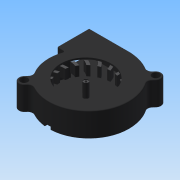
# Autodesk Inventor part: 5015 kuler obduva ulitla
Saved by Autodesk Inventor 2017 (Build 210142000, 142)
## iProperties
Part Number: 5015 kuler obduva ulitla
Material: Типовые
Document SubType Name: Modeling
Designer: alcapone
Density: 1 g/cm^3
Appearance: Резина — черная
Mass: 8.81297 g
Surface Area: 142.043 cm^2
Volume: 8.81297 cm^3
Author: alcapone
Autodesk Inventor part; units mm, degrees
ref_plane "YZ Plane" through (0, 0, 0) normal (1, 0, 0) x (0, 1, 0)
ref_plane "XZ Plane" through (0, 0, 0) normal (0, 1, 0) x (-1, 0, 0)
ref_plane "XY Plane" through (0, 0, 0) normal (0, 0, 1) x (1, 0, 0)
sketch "Эскиз1" plane through (0, 0, 0) normal (0, 0, 1) x (1, 0, 0)
  circle A0 centre (0, 0) radius 13
  circle A1 centre (0, 0) radius 15.5
  circle A2 centre (-18, -20) radius 2.25
  circle A3 centre (20, 23) radius 2.25
  line L0 (-25.4, 27.55) -> (-25.4, 7.95)
  line L1 (-25.4, 7.95) -> (-22, 7.95)
  line L2 (-25.4, 27.55) -> (0, 27.55)
  line L3 (25.6, 31.451287) -> (25.6, -25.798713) construction
  arc A4 (22.43532, 20.847857) -> (17.56468, 25.152143) centre (20, 23) ccw
  arc A5 (-20.43532, -17.847857) -> (-15.56468, -22.152143) centre (-18, -20) ccw
  line L4 (17.56468, 25.152143) -> (16.739143, 24.217982)
  line L5 (-19.151802, -16.395455) -> (-20.43532, -17.847857)
  line L6 (21.282046, 19.542837) -> (22.43532, 20.847857)
  line L7 (-15.56468, -22.152143) -> (-14.81527, -21.304126)
  line L8 (-54, -23.75) -> (48, -23.75) construction
  arc A6 (-11.116766, -20.664695) -> (25.6, 1) centre (0.85, 1) ccw
  arc A7 (-21.05304, 6.62865) -> (-18.846796, -12.833353) centre (0.718164, -0.759385) ccw
  arc A8 (-21.05304, 6.62865) -> (-22, 7.95) centre (-22, 6.95) ccw
  arc A9 (-19.151802, -16.395455) -> (-18.846796, -12.833353) centre (-21.399789, -14.408862) ccw
  arc A10 (-11.116766, -20.664695) -> (-14.81527, -21.304126) centre (-12.567283, -23.290719) ccw
  arc A11 (25.6, 1) -> (21.044444, 15.876409) centre (-0.967627, 1) ccw
  arc A12 (12.922672, 23.64726) -> (0, 27.55) centre (-0.967627, 1) ccw
  arc A13 (12.922672, 23.64726) -> (16.739143, 24.217982) centre (14.491156, 26.204575) ccw
  arc A14 (21.282046, 19.542837) -> (21.044444, 15.876409) centre (23.530033, 17.556244) ccw
  line L9 (-25.4, 26.2) -> (1.943816, 26.2)
  line L10 (-25.4, 9.3) -> (-18.611597, 9.3)
  arc A15 (-18.611597, 9.3) -> (0.782803, -22.549904) centre (0.718164, -0.759385) ccw
  arc A16 (0.782803, -22.549904) -> (24.4, 1) centre (0.85, 1) ccw
  arc A17 (24.4, 1) -> (1.943816, 26.2) centre (-0.967627, 1) ccw
  line L11 (-25.4, 27.55) -> (-25.4, 26.2)
  line L12 (-25.4, 9.3) -> (-25.4, 7.95)
  point P0 (-20.558936, 7.95)
  point P1 (14.991388, 22.24026)
  point P2 (-17.605238, -14.645396)
  point P3 (19.675218, 17.724585)
  point P4 (-13.144564, -19.41359)
  dimension "d0" = 26
  dimension "d1" = 31
  dimension "d2" = 4.5
  dimension "d3" = 4.5
  dimension "d4" = 20
  dimension "d5" = 18
  dimension "d6" = 20
  dimension "d7" = 23
  dimension "d8" = 25.4
  dimension "d9" = 25.4
  dimension "d10" = 51
  dimension "d12" = 19.6
  dimension "d13" = 6.5
  dimension "d14" = 6.5
  dimension "d16" = 25.6
  dimension "d17" = 51.3
  dimension "d18" = 0.5
  dimension "d19" = 1
  dimension "d20" = 22
  dimension "d21" = 3
  dimension "d22" = 3
  dimension "d23" = 22.99062
  dimension "d24" = 24.75
  dimension "d25" = 3
  dimension "d26" = 26.56763
  dimension "d27" = 26.56763
  dimension "d28" = 1.35
  dimension "d29" = 1.35
  dimension "d30" = 1.2
  dimension "d31" = 1.2
  dimension "d32" = 1.2
  dimension "d133" = 90
  dimension "d138" = 16.9
  constraints: 33 point on circle, 26 end point, 20 tangent, 18 centre point, 8 point on line, 7 coincident, 3 parallel, 2 collinear, 2 horizontal, 2 perpendicular, 2 vertical, 1 equal radius
  measures "d0" diameter of A0
  measures "d1" diameter of A1
  measures "d2" diameter of A2
  measures "d3" diameter of A3
  measures "d4" vertical distance of A2.centre A1.centre
  measures "d5" horizontal distance of point (0, 0) A2.centre
  measures "d6" horizontal distance of point (0, 0) A3.centre
  measures "d7" vertical distance of A3.centre point (0, 0)
  measures "d8" distance from line of point (0, 0) L0
  measures "d9" distance of L0.start L2.end
  measures "d10" distance between parallel lines of L0 L3
  measures "d12" distance between parallel lines of L1 L2
  measures "d13" diameter of A4
  measures "d14" diameter of A5
  measures "d16" distance from line of L3 point (0, 0)
  measures "d17" distance between parallel lines of L8 L2
  measures "d18" distance edge to line of A5 L8
  measures "d19" radius of A8
  measures "d20" horizontal distance of point (0, 0) A8.centre
  measures "d21" radius of A9
  measures "d22" radius of A10
  measures "d23" radius of A7
  measures "d24" radius of A6
  measures "d25" radius of A13
  measures "d26" radius of A12
  measures "d27" radius of A11
  measures "d28" distance between parallel lines of L9 L2
  measures "d29" distance between parallel lines of L10 L1
  measures "d30" radial gap between concentric circles of A7 A15
  measures "d31" radial gap between concentric circles of A6 A16
  measures "d32" radial gap between concentric circles of A12 A17
  measures "d133" angle of L2 L0
  measures "d138" distance between parallel lines of L10 L9
sketch "Эскиз1 outline for Выдавливание1" plane through (0, 0, 0) normal (0, 0, 1) x (1, 0, 0)
  line L0 (0, 27.55) -> (-25.4, 27.55)
  line L1 (-25.4, 27.55) -> (-25.4, 7.95)
  line L2 (-25.4, 7.95) -> (-22, 7.95)
  arc A0 (-22, 7.95) -> (-21.05304, 6.62865) centre (-22, 6.95) cw
  arc A1 (-21.05304, 6.62865) -> (-18.846796, -12.833353) centre (0.718164, -0.759385) ccw
  arc A2 (-18.846796, -12.833353) -> (-19.151802, -16.395455) centre (-21.399789, -14.408862) cw
  line L3 (-19.151802, -16.395455) -> (-20.43532, -17.847857)
  arc A3 (-20.43532, -17.847857) -> (-15.56468, -22.152143) centre (-18, -20) ccw
  line L4 (-15.56468, -22.152143) -> (-14.81527, -21.304126)
  arc A4 (-14.81527, -21.304126) -> (-11.116766, -20.664695) centre (-12.567283, -23.290719) cw
  arc A5 (-11.116766, -20.664695) -> (25.6, 1) centre (0.85, 1) ccw
  arc A6 (25.6, 1) -> (21.044444, 15.876409) centre (-0.967627, 1) ccw
  arc A7 (21.044444, 15.876409) -> (21.282046, 19.542837) centre (23.530033, 17.556244) cw
  line L5 (21.282046, 19.542837) -> (22.43532, 20.847857)
  arc A8 (22.43532, 20.847857) -> (17.56468, 25.152143) centre (20, 23) ccw
  line L6 (17.56468, 25.152143) -> (16.739143, 24.217982)
  arc A9 (16.739143, 24.217982) -> (12.922672, 23.64726) centre (14.491156, 26.204575) cw
  arc A10 (12.922672, 23.64726) -> (0, 27.55) centre (-0.967627, 1) ccw
  circle A11 centre (-18, -20) radius 2.25
  circle A12 centre (20, 23) radius 2.25
  circle A13 centre (0, 0) radius 15.5
extrude "Выдавливание1" add sketch "Эскиз1 outline for Выдавливание1" along normal mid plane 15
sketch "Эскиз1 outline for Выдавливание2" plane through (0, 0, 0) normal (0, 0, 1) x (1, 0, 0)
  circle A0 centre (0, 0) radius 15.5
extrude "Выдавливание2" add sketch "Эскиз1 outline for Выдавливание2" against normal blind 7.5
sketch "Эскиз1 outline for Выдавливание3" plane through (0, 0, 0) normal (0, 0, 1) x (1, 0, 0)
  line L0 (1.943816, 26.2) -> (-25.4, 26.2)
  arc A0 (24.4, 1) -> (1.943816, 26.2) centre (-0.967627, 1) ccw
  arc A1 (0.782803, -22.549904) -> (24.4, 1) centre (0.85, 1) ccw
  arc A2 (-18.611597, 9.3) -> (0.782803, -22.549904) centre (0.718164, -0.759385) ccw
  line L1 (-25.4, 9.3) -> (-18.611597, 9.3)
  line L2 (-25.4, 26.2) -> (-25.4, 9.3)
extrude "Выдавливание3" cut sketch "Эскиз1 outline for Выдавливание3" along normal blind 6.5 and the other way blind 6.2
sketch "Эскиз2" plane through (0, 0, -7.5) normal (0, 0, -1) x (-1, 0, 0)
  line L0 (0, 0) -> (0, 39) construction
  arc A0 (2, -8.774964) -> (-2, -8.774964) centre (0, 0) ccw
  arc A1 (-1.943816, 26.2) -> (-24.4, 1) centre (0.967627, 1) ccw
  arc A2 (-24.4, 1) -> (-0.782803, -22.549904) centre (-0.85, 1) ccw
  arc A3 (-0.782803, -22.549904) -> (18.611597, 9.3) centre (-0.718164, -0.759385) ccw
  arc A4 (-22.887217, 9.629191) -> (-24.4, 1) centre (0.967627, 1) ccw
  line L1 (-2, -20) -> (1, -20)
  line L2 (1, -20) -> (1, -18.276492)
  line L3 (1, -18.276492) -> (-2, -18.276492)
  line L4 (-3, -22.451652) -> (-3, -9.539392)
  line L5 (3, -9.539392) -> (3, -22.230439)
  line L6 (-2, -8.774964) -> (-2, -18.276492)
  line L7 (-2, -20) -> (-2, -22.521905)
  line L8 (2, -22.379803) -> (2, -8.774964)
  arc A5 (-2, -22.521905) -> (2, -22.376912) centre (-0.85, 1) ccw
  line L9 (-0.8, 9.967949) -> (-0.8, 24.420616)
  line L10 (0.8, 24.293495) -> (0.8, 9.967949)
  line L11 (0, 0) -> (-32, 0) construction
  line L12 (0, 0) -> (28, 0) construction
  line L13 (0, 0.533734) -> (-31.257467, 31.7912) construction
  line L14 (0, 0) -> (-29.841247, -29.841247) construction
  arc A6 (-0.8, 9.967949) -> (-6.189332, 7.854436) centre (0, 0) ccw
  line L15 (-24.399212, 0.8) -> (-9.967949, 0.8)
  line L16 (-9.967949, -0.8) -> (-24.331109, -0.8)
  line L17 (9.967949, 0.8) -> (21.028696, 0.8)
  line L18 (10.072158, -0.8) -> (21.072413, -0.8)
  line L19 (6.482719, 7.614089) -> (15.385181, 16.516552)
  line L20 (-15.944824, -17.076194) -> (-6.482719, -7.614089)
  line L21 (7.614089, 6.482719) -> (16.394183, 15.262812)
  arc A7 (9.967949, 0.8) -> (7.614089, 6.482719) centre (0, 0) ccw
  arc A8 (6.482719, 7.614089) -> (0.8, 9.967949) centre (0, 0) ccw
  arc A9 (-6.482719, -7.614089) -> (-3, -9.539392) centre (0, 0) ccw
  arc A10 (-7.36357, 6.765932) -> (-9.967949, 0.8) centre (0, 0) ccw
  arc A11 (-9.967949, -0.8) -> (-7.614089, -6.482719) centre (0, 0) ccw
  line L22 (-17.139173, -16.007802) -> (-7.614089, -6.482719)
  arc A12 (3, -9.539392) -> (6.765932, -7.36357) centre (0, 0) ccw
  arc A13 (7.986272, -6.189332) -> (10.072158, -0.8) centre (0, 0) ccw
  line L23 (-16.909631, 18.574735) -> (-6.189332, 7.854436)
  line L24 (7.986272, -6.189332) -> (16.24014, -14.4432)
  line L25 (15.123801, -15.721438) -> (6.765932, -7.36357)
  line L26 (-7.36357, 6.765932) -> (-18.052335, 17.454698)
  arc A14 (-18.052335, 17.454698) -> (-22.887217, 9.629191) centre (-1.776858, 1.992783) ccw
  arc A15 (10.33458, 20.894503) -> (0.8, 24.293495) centre (-1.776858, 1.992783) ccw
  arc A16 (-0.8, 24.420616) -> (-16.909631, 18.574735) centre (-1.776858, 1.992783) ccw
  arc A17 (21.028696, 0.8) -> (10.33458, 20.894503) centre (-2.20156, 1.329972) ccw
  arc A18 (3, -22.230439) -> (15.123801, -15.721438) centre (-0.718164, -0.759385) ccw
  arc A19 (16.24014, -14.4432) -> (21.072451, -0.759385) centre (-0.718164, -0.759385) ccw
  arc A20 (-15.944824, -17.076194) -> (-3, -22.451652) centre (-0.85, 1) ccw
  arc A21 (-24.331109, -0.8) -> (-17.139173, -16.007802) centre (-0.85, 1) ccw
  line L27 (-24.4, 1) -> (-24.399212, 0.8)
  dimension "d42" = 3
  dimension "d43" = 4
  dimension "d45" = 1
  dimension "d46" = 1
  dimension "d49" = 45
  dimension "d50" = 45
  dimension "d52" = 1.6
  dimension "d53" = 1.6
  dimension "d54" = 10
  dimension "d59" = 10
  dimension "d60" = 10
  dimension "d61" = 10
  dimension "d62" = 10
  dimension "d63" = 9
  dimension "d64" = 1.6
  dimension "d66" = 0.8
  dimension "d67" = 0.8
  constraints: 56 end point, 54 point on circle, 19 centre point, 10 parallel, 3 horizontal, 3 vertical, 2 coincident, 2 perpendicular, 2 point on line, 1 concentric, 7 other
  measures "d42" distance between parallel lines of L0 L4
  measures "d43" distance between parallel lines of L4 L2
  measures "d45" distance between parallel lines of L4 L6
  measures "d46" distance between parallel lines of L5 L8
  measures "d49" angle of L11 L13
  measures "d50" angle of L11 L14
  measures "d52" distance between parallel lines of L16 L15
  measures "d53" distance between parallel lines of L18 L17
  measures "d54" radius of A6
  measures "d59" radius of A10
  measures "d60" radius of A11
  measures "d61" radius of A8
  measures "d62" radius of A7
  measures "d63" radius of A0
  measures "d64" distance between parallel lines of L21 L19
  measures "d66" distance between parallel lines of L20 L14
  measures "d67" distance between parallel lines of L14 L22
sketch "Эскиз2 outline for Выдавливание4" plane through (0, 0, -7.5) normal (0, 0, -1) x (-1, 0, 0)
  line L0 (3, -9.539392) -> (3, -22.230439)
  arc A0 (6.765932, -7.36357) -> (3, -9.539392) centre (0, 0) cw
  line L1 (15.123801, -15.721438) -> (6.765932, -7.36357)
  arc A1 (3, -22.230439) -> (15.123801, -15.721438) centre (-0.718164, -0.759385) ccw
  arc A2 (16.24014, -14.4432) -> (21.072413, -0.8) centre (-0.718164, -0.759385) ccw
  line L2 (7.986272, -6.189332) -> (16.24014, -14.4432)
  arc A3 (10.072158, -0.8) -> (7.986272, -6.189332) centre (0, 0) cw
  line L3 (21.072413, -0.8) -> (10.072158, -0.8)
  line L4 (-6.482719, -7.614089) -> (-15.944824, -17.076194)
  arc A4 (-3, -9.539392) -> (-6.482719, -7.614089) centre (0, 0) cw
  line L5 (-3, -22.451652) -> (-3, -9.539392)
  arc A5 (-15.944824, -17.076194) -> (-3, -22.451652) centre (-0.85, 1) ccw
  arc A6 (21.028696, 0.8) -> (16.394183, 15.262812) centre (-2.20156, 1.329972) ccw
  line L6 (9.967949, 0.8) -> (21.028696, 0.8)
  arc A7 (7.614089, 6.482719) -> (9.967949, 0.8) centre (0, 0) cw
  line L7 (16.394183, 15.262812) -> (7.614089, 6.482719)
  arc A8 (15.385181, 16.516552) -> (10.33458, 20.894503) centre (-2.20156, 1.329972) ccw
  line L8 (6.482719, 7.614089) -> (15.385181, 16.516552)
  arc A9 (0.8, 9.967949) -> (6.482719, 7.614089) centre (0, 0) cw
  line L9 (0.8, 24.293495) -> (0.8, 9.967949)
  arc A10 (10.33458, 20.894503) -> (0.8, 24.293495) centre (-1.776858, 1.992783) ccw
  line L10 (-9.967949, -0.8) -> (-24.331109, -0.8)
  arc A11 (-7.614089, -6.482719) -> (-9.967949, -0.8) centre (0, 0) cw
  line L11 (-17.139173, -16.007802) -> (-7.614089, -6.482719)
  arc A12 (-24.331109, -0.8) -> (-17.139173, -16.007802) centre (-0.85, 1) ccw
  line L12 (-0.8, 24.420616) -> (-0.8, 9.967949)
  arc A13 (-0.8, 9.967949) -> (-6.189332, 7.854436) centre (0, 0) ccw
  line L13 (-6.189332, 7.854436) -> (-16.909631, 18.574735)
  arc A14 (-16.909631, 18.574735) -> (-0.8, 24.420616) centre (-1.776858, 1.992783) cw
  arc A15 (-22.887217, 9.629191) -> (-24.4, 1) centre (0.967627, 1) ccw
  arc A16 (-18.052335, 17.454698) -> (-22.887217, 9.629191) centre (-1.776858, 1.992783) ccw
  line L14 (-7.36357, 6.765932) -> (-18.052335, 17.454698)
  arc A17 (-9.967949, 0.8) -> (-7.36357, 6.765932) centre (0, 0) cw
  line L15 (-24.399212, 0.8) -> (-9.967949, 0.8)
  line L16 (-24.4, 1) -> (-24.399212, 0.8)
extrude "Выдавливание4" cut sketch "Эскиз2 outline for Выдавливание4" against normal blind 0.5
sketch "Эскиз3" plane through (0, 0, -7.5) normal (0, 0, -1) x (-1, 0, 0)
  arc A0 (3, -9.539392) -> (-3, -9.539392) centre (0, 0) ccw
  line L0 (-3, -9.539392) -> (-3, -22.451652)
  arc A1 (-25.6, 1) -> (11.116766, -20.664695) centre (-0.85, 1) ccw
  line L1 (3, -9.539392) -> (2.99982, -9.539392)
  line L2 (2.99982, -9.539392) -> (2.99982, -23.44875)
  line L3 (-3, -23.656439) -> (-3, -9.539392)
  arc A2 (-3, -23.656439) -> (2.99982, -23.44875) centre (-0.85, 1) ccw
  constraints: 6 end point, 6 point on circle, 2 centre point, 1 coincident, 1 concentric, 1 horizontal, 1 parallel, 1 perpendicular
sketch "Эскиз3 outline for Выдавливание5" plane through (0, 0, -7.5) normal (0, 0, -1) x (-1, 0, 0)
  arc A0 (2.99982, -9.539392) -> (-3, -9.539392) centre (-0.00009, 0.000014) ccw
  line L0 (2.99982, -23.44875) -> (2.99982, -9.539392)
  arc A1 (-3, -23.656439) -> (2.99982, -23.44875) centre (-0.85, 1) ccw
  line L1 (-3, -9.539392) -> (-3, -23.656439)
extrude "Выдавливание5" add sketch "Эскиз3 outline for Выдавливание5" against normal blind 5
sketch "Эскиз2 outline for Выдавливание6" plane through (0, 0, -7.5) normal (0, 0, -1) x (-1, 0, 0)
  line L0 (-2, -20) -> (-2, -22.521905)
  line L1 (1, -20) -> (-2, -20)
  line L2 (1, -18.276492) -> (1, -20)
  line L3 (-2, -18.276492) -> (1, -18.276492)
  line L4 (-2, -8.774964) -> (-2, -18.276492)
  arc A0 (2, -8.774964) -> (-2, -8.774964) centre (0, 0) ccw
  line L5 (2, -22.379803) -> (2, -8.774964)
  arc A1 (-0.782803, -22.549904) -> (2, -22.379803) centre (-0.718164, -0.759385) ccw
  arc A2 (-2, -22.521905) -> (-0.782803, -22.549904) centre (-0.85, 1) ccw
extrude "Выдавливание6" cut sketch "Эскиз2 outline for Выдавливание6" against normal blind 4
sketch "Эскиз4" plane through (0, 0, -3.5) normal (0, 0, -1) x (-1, 0, 0)
  circle A0 centre (0, 0) radius 9
  constraints: 1 centre point, 1 coincident
sketch "Эскиз4 outline for Выдавливание7" plane through (0, 0, -3.5) normal (0, 0, -1) x (-1, 0, 0)
  circle A0 centre (0, 0) radius 9
extrude "Выдавливание7" add sketch "Эскиз4 outline for Выдавливание7" along normal blind 3.5
sketch "Эскиз5" plane through (0, 0, -7) normal (0, 0, -1) x (-1, 0, 0)
  circle A0 centre (0, 0) radius 15.5
  line L0 (12.267038, 9.474692) -> (8.945531, -12.658099) construction
  line L1 (8.945531, -12.658099) -> (-12.429289, -9.450342) construction
  line L2 (-12.429289, -9.450342) -> (-9.107783, 12.682448) construction
  line L3 (-9.107783, 12.682448) -> (12.267038, 9.474692) construction
  constraints: 2 point on circle, 2 other
decal "Маркировка1"
sketch "Эскиз6" plane through (0, 0, -7.5) normal (0, 0, -1) x (-1, 0, 0)
  line L0 (-2, -22.521905) -> (-2, -20)
  line L1 (-2, -22) -> (-2, -23.723268)
  arc A0 (-25.6, 1) -> (11.116766, -20.664695) centre (-0.85, 1) ccw
  arc A1 (-2, -23.723268) -> (2, -23.585361) centre (-0.85, 1) ccw
  line L2 (2, -8.774964) -> (2, -22.379803)
  line L3 (2, -22) -> (2, -23.585361)
  arc A2 (-2, -22) -> (2, -22) centre (0, -16.721398) ccw
  point P0 (0, 0)
  constraints: 6 point on circle, 4 end point, 2 centre point, 2 concentric, 1 collinear, 1 vertical
sketch "Эскиз6 outline for Выдавливание8" plane through (0, 0, -7.5) normal (0, 0, -1) x (-1, 0, 0)
  line L0 (-2, -22) -> (-2, -23.723268)
  arc A0 (2, -22) -> (-2, -22) centre (0, -16.721398) cw
  line L1 (2, -23.585361) -> (2, -22)
  arc A1 (-2, -23.723268) -> (2, -23.585361) centre (-0.85, 1) ccw
extrude "Выдавливание8" cut sketch "Эскиз6 outline for Выдавливание8" against normal blind 2
sketch "Эскиз7" plane through (0, 0, -2.5) normal (0, 0, 1) x (1, 0, 0)
  circle A0 centre (0, 0) radius 13
  arc A1 (0, 13) -> (-2, 19) centre (-14.5, 11.5) ccw
  line L0 (-2, 19) -> (-4, 19)
  arc A2 (-2, 12.845233) -> (-4, 19) centre (-11.85714, 13.044477) ccw
  dimension "d103" = 2
  dimension "d104" = 26
  dimension "d105" = 2
  constraints: 6 point on circle, 3 centre point, 2 end point, 1 coincident
  measures "d103" horizontal distance of A0.start A0.end
  measures "d104" diameter of A0
  measures "d105" distance of L0.start L0.end
sketch "Эскиз7 outline for Выдавливание9" plane through (0, 0, -2.5) normal (0, 0, 1) x (1, 0, 0)
  arc A0 (-2, 12.845233) -> (0, 13) centre (0, 0) cw
  arc A1 (-4, 19) -> (-2, 12.845233) centre (-11.85714, 13.044477) cw
  line L0 (-2, 19) -> (-4, 19)
  arc A2 (0, 13) -> (-2, 19) centre (-14.5, 11.5) ccw
extrude "Выдавливание9" add sketch "Эскиз7 outline for Выдавливание9" along normal blind 6
sketch "Эскиз7 outline for Выдавливание10" plane through (0, 0, -2.5) normal (0, 0, 1) x (1, 0, 0)
  arc A0 (-2, 12.845233) -> (0, 13) centre (0, 0) ccw
  arc A1 (0, 13) -> (-2, 12.845233) centre (0, 0) ccw
extrude "Выдавливание10" add sketch "Эскиз7 outline for Выдавливание10" along normal blind 8.5
pattern_circular "Круговой массив1" count 20 over 360 about axis through (0, 0, -2.5) along (0, 0, 1) of "Выдавливание9"
fillet "Сопряжение1" radius 1 1 edges at (0, -13, 6)
sketch "Эскиз8" plane through (0, 0, 6) normal (0, 0, 1) x (1, 0, 0)
  circle A0 centre (0, 0) radius 1.5
  circle A1 centre (0, 0) radius 0.5
  dimension "d114" = 1
  dimension "d115" = 3
  constraints: 2 centre point, 2 coincident
  measures "d114" diameter of A1
  measures "d115" diameter of A0
sketch "Эскиз8 outline for Выдавливание11" plane through (0, 0, 6) normal (0, 0, 1) x (1, 0, 0)
  circle A0 centre (0, 0) radius 1.5
  circle A1 centre (0, 0) radius 0.5
extrude "Выдавливание11" cut sketch "Эскиз8 outline for Выдавливание11" against normal blind 0.5
fillet "Сопряжение2" radius 0.5 35 edges at (-12.7, 27.55, -7.5) (-12.7, 27.55, 7.5) (14.9348, 23.2376, -7.5) (17.1519, 24.6851, -7.5) (22.1521, 25.4353, -7.5) (21.8587, 20.1953, -7.5) (20.5363, 17.7503, -7.5) (24.4356, 8.7791, -7.5) (18.7529, -16.0895, -7.5) (6.7133, 26.4331, -7.5) (6.7133, 26.4331, 7.5) (17.1519, 24.6851, 7.5) (22.1521, 25.4353, 7.5) (21.8587, 20.1953, 7.5) (20.5363, 17.7503, 7.5) (24.4356, 8.7791, 7.5) (13.4275, -20.316, 7.5) (-13.0784, -20.3346, 7.5) (-15.19, -21.7281, 7.5) (-20.1521, -22.4353, 7.5) (-19.7936, -17.1217, 7.5) (-18.4107, -14.6648, 7.5) (-22.1261, -3.3491, 7.5) (-21.1872, 7.5325, 7.5) (-23.7, 7.95, 7.5) (14.9348, 23.2376, 7.5) (-13.0784, -20.3346, -7.5) (-15.19, -21.7281, -7.5) (-20.1521, -22.4353, -7.5) (-19.7936, -17.1217, -7.5) (-18.4107, -14.6648, -7.5) (-22.1261, -3.3491, -7.5) (-21.1872, 7.5325, -7.5) (-23.7, 7.95, -7.5) (-6.7009, -22.57, -7.5)
fillet "Сопряжение3" radius 0.2 8 edges at (-25.4, 27.4036, -7.3536) (-25.4, 17.75, -7.5) (-25.4, 8.0964, -7.3536) (-25.4, 7.95, 0) (-25.4, 8.0964, 7.3536) (-25.4, 17.75, 7.5) (-25.4, 27.4036, 7.3536) (-25.4, 27.55, 0)
sketch "Эскиз9" plane through (0, 27.55, 7) normal (0, 1, 0) x (1, 0, 0)
  line L0 (0, 7) -> (-25.2, 7) construction
  line L1 (-25.2, 14) -> (-25.2, 0) construction
  line L2 (-13.55, 5.75) -> (-22.05, 5.75)
  line L3 (-22.05, 5.75) -> (-22.05, 8.25)
  line L4 (-22.05, 8.25) -> (-13.55, 8.25)
  line L5 (-13.55, 8.25) -> (-13.55, 5.75)
  line L6 (-25.4, 14) -> (-25.4, 0) projected
  dimension "d120" = 2.5
  dimension "d121" = 11.85
  dimension "d122" = 8.5
  constraints: 10 end point, 2 parallel, 1 horizontal, 1 midpoint, 1 perpendicular, 1 other
  measures "d120" distance between parallel lines of L4 L2
  measures "d121" distance between parallel lines of L6 L5
  measures "d122" distance between parallel lines of L3 L5
sketch "Эскиз9 outline for Выдавливание12" plane through (0, 27.55, 7) normal (0, 1, 0) x (1, 0, 0)
  line L0 (-13.55, 5.75) -> (-22.05, 5.75)
  line L1 (-22.05, 5.75) -> (-22.05, 8.25)
  line L2 (-22.05, 8.25) -> (-13.55, 8.25)
  line L3 (-13.55, 8.25) -> (-13.55, 5.75)
extrude "Выдавливание12" add sketch "Эскиз9 outline for Выдавливание12" along normal blind 1
fillet "Сопряжение4" radius 0.5 2 edges at (-17.8, 28.55, 1.25) (-17.8, 28.55, -1.25)
sketch "Эскиз10" plane through (0, 0, 0) normal (0, 0, 1) x (1, 0, 0)
  arc A0 (-21.05304, 6.62865) -> (-18.846796, -12.833353) centre (0.718164, -0.759385) ccw
  arc A1 (-20.579559, 6.467975) -> (-18.421297, -12.570769) centre (0.718164, -0.759385) ccw
  arc A2 (-22.650984, 4.55) -> (-23.033186, -3.95) centre (0.718164, -0.759385) ccw
  line L0 (-22.650984, 4.55) -> (-21.650984, 4.55)
  arc A3 (-21.05304, 6.62865) -> (-18.846796, -12.833353) centre (0.718164, -0.759385) ccw
  line L1 (-22.049979, -3.95) -> (-23.033186, -3.95)
  line L2 (-22, 7.95) -> (-25.2, 7.95)
  point P0 (0, 0)
  dimension "d126" = 22.99062
  dimension "d127" = 3.4
  dimension "d128" = 8.5
  dimension "d129" = 1
  constraints: 6 point on circle, 4 end point, 1 centre point, 1 coincident, 1 horizontal, 1 parallel
  measures "d126" radius of A0
  measures "d127" distance between parallel lines of L0 L2
  measures "d128" distance between parallel lines of L1 L0
  measures "d129" distance of L0.start L0.end
sketch "Эскиз10 outline for Выдавливание13" plane through (0, 0, 0) normal (0, 0, 1) x (1, 0, 0)
  line L0 (-23.033186, -3.95) -> (-22.049979, -3.95)
  arc A0 (-22.650984, 4.55) -> (-23.033186, -3.95) centre (0.718164, -0.759385) ccw
  line L1 (-21.650984, 4.55) -> (-22.650984, 4.55)
  arc A1 (-22.049979, -3.95) -> (-21.650984, 4.55) centre (0.718164, -0.759385) cw
extrude "Выдавливание13" add sketch "Эскиз10 outline for Выдавливание13" along normal mid plane 2.5
fillet "Сопряжение5" radius 0.5 2 edges at (-23.2223, 0.3171, -1.25) (-23.2223, 0.3171, 1.25)
sketch "Эскиз12" plane through (0, 0, 7.5) normal (0, 0, 1) x (1, 0, 0)
  circle A0 centre (0, 0) radius 1.5
  circle A1 centre (0, 0) radius 15.5
  circle A2 centre (0, 0) radius 0.5
  circle A3 centre (0, 0) radius 1.568896
  constraints: 2 centre point, 2 coincident
sketch "Эскиз12 outline for Выдавливание14" plane through (0, 0, 7.5) normal (0, 0, 1) x (1, 0, 0)
  circle A0 centre (0, 0) radius 15.5
  circle A1 centre (0, 0) radius 1.568896
extrude "Выдавливание14" cut sketch "Эскиз12 outline for Выдавливание14" against normal blind 10
